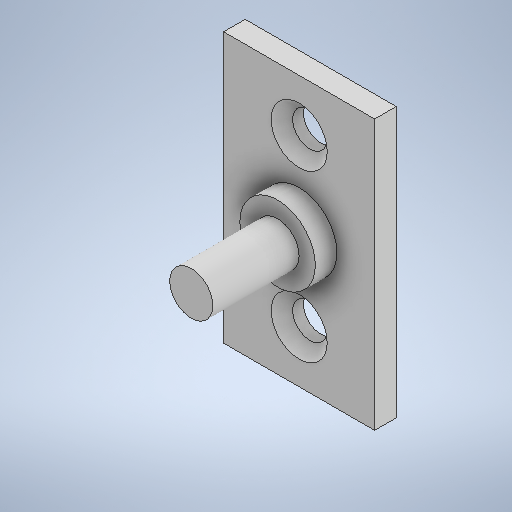
# Autodesk Inventor part: BearingMount-ExtrusionBtm
Saved by Autodesk Inventor 2025.2 (Build 292293000, 293)
## iProperties
Created: 2025-01-10
Part Number: BearingMount-ExtrusionBtm
Material: Generic
Document SubType Name: Modeling
Designer: dcfam
Density: 1 g/cm^3
Appearance: Default
Author: dcfam
Autodesk Inventor part; units mm, degrees
ref_plane "YZ Plane" through (0, 0, 0) normal (1, 0, 0) x (0, 1, 0)
ref_plane "XZ Plane" through (0, 0, 0) normal (0, 1, 0) x (-1, 0, 0)
ref_plane "XY Plane" through (0, 0, 0) normal (0, 0, 1) x (1, 0, 0)
sketch "Sketch1" plane through (0, 0, 0) normal (0, 0, 1) x (1, 0, 0)
  line L0 (-7, -12.5) -> (7, -12.5)
  line L1 (7, -12.5) -> (7, 12.5)
  line L2 (7, 12.5) -> (-7, 12.5)
  line L3 (-7, 12.5) -> (-7, -12.5)
  line L4 (-7, -12.5) -> (7, 12.5) construction
  line L5 (7, -12.5) -> (-7, 12.5) construction
  point P0 (0, 0)
  dimension "d0" = 14
  dimension "d1" = 25
  constraints: 12 end point, 2 midpoint, 2 parallel, 1 horizontal, 1 perpendicular
  measures "d0" distance of L2.end L1.end
  measures "d1" distance of L1.end L0.end
extrude "Extrusion1" add sketch "Sketch1" along normal blind 2
sketch "Sketch2" plane through (0, 0, 2) normal (0, 0, 1) x (1, 0, 0)
  circle A0 centre (0, 7.6788) radius 1.6
  line L0 (-7, 12.5) -> (-7, -12.5) construction
  line L1 (-7, 0) -> (7, 0) construction
  line L2 (7, -12.5) -> (7, 12.5) construction
  circle A1 centre (0, -7.6788) radius 1.6
  point P0 (0, 0)
  dimension "d4" = 3.2
  constraints: 2 centre point, 2 end point, 2 midpoint, 1 symmetric about line, 1 other
  measures "d4" diameter of A0
extrude "Extrusion2" cut sketch "Sketch2" against normal blind 2
sketch "Sketch3" plane through (0, 0, 2) normal (0, 0, 1) x (1, 0, 0)
  circle A0 centre (0, 0) radius 2
  dimension "d7" = 4
  constraints: 1 centre point, 1 coincident
  measures "d7" diameter of A0
extrude "Extrusion3" add sketch "Sketch3" along normal blind 10
sketch "Sketch4" plane through (0, 0, 2) normal (0, 0, 1) x (1, 0, 0)
  circle A0 centre (0, 0) radius 2 projected
  circle A1 centre (0, 0) radius 3.5
  dimension "d10" = 1.5
  constraints: 1 centre point
  measures "d10" radial gap between concentric circles of A0 A1
extrude "Extrusion4" add sketch "Sketch4" along normal blind 2
chamfer "Chamfer1" distance 1 angle 45 2 edges at (-1.6, -7.6788, 2) (-1.6, 7.6788, 2)
body "Solid1"
